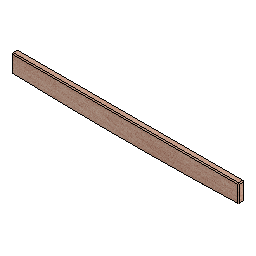
model (Autodesk Fusion 360 design; units mm, degrees)
Autodesk Fusion 360 part; units mm, degrees
sketch "Sketch1" plane through (0, 0, 0) normal (0, 1, 0) x (1, 0, 0)
  line L0 (0, 0) -> (0, -42.45) construction
  line L1 (0, -42.45) -> (480, -42.45)
  line L2 (480, -42.45) -> (480, 0) construction
  line L3 (480, 0) -> (0, 0) construction
  line L4 (0, -42.45) -> (0, -4)
  line L5 (480, -42.45) -> (480, -4)
  arc A0 (480, -4) -> (0, -4) centre (240, -7202) ccw
  dimension "d1" = 480
  dimension "d2" = 4
  dimension "d3" = 42.45
  constraint coincident L0.start L3.end
  constraint vertical L0
  constraint vertical L2
  constraint horizontal L3
  constraint horizontal L1
  constraint coincident L0 L4.end
  constraint perpendicular L1 L4
  constraint coincident L2 L5.end
  constraint tangent L3 A0
  constraint equal L4 L5
  measures "d1" distance of L2.end L0.start
  measures "d2" distance of L0.start L4.end
  measures "d3" distance of L0.start L0.end
extrude "Extrude1" add sketch "Sketch1" along normal blind 13
chamfer "Chamfer1" distance 2 angle 45 10 edges at (240, 0, 0) (0, 0, 23.225) (0, 6.5, 42.45) (480, 0, 23.225) (480, 6.5, 4) (0, 13, 23.225) (240, 0, 42.45) (480, 6.5, 42.45) (240, 13, 42.45) (480, 13, 23.225) 4 faces at (213.3289, 13, 28.4482) (480, 4.3333, 29.6333) (213.3289, 0, 28.4482) (160, 4.3333, 42.45)
equation "d3 = 1.75 in - 2 mm"
